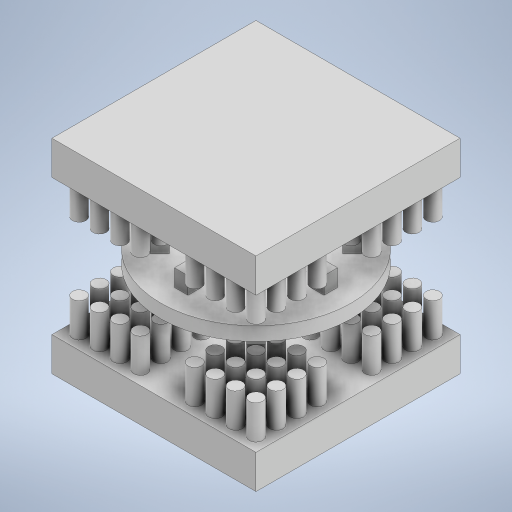
# Autodesk Inventor part: Part2
Saved by Autodesk Inventor 2024 (Build 280153000, 153)
## iProperties
Created: 2023-04-21
Part Number: Part2
Material: Generic
Document SubType Name: Modeling
Designer: Raj
Density: 1 g/cm^3
Appearance: Default
Author: Raj
Autodesk Inventor part; units mm, degrees
ref_plane "YZ Plane" through (0, 0, 0) normal (1, 0, 0) x (0, 1, 0)
ref_plane "XZ Plane" through (0, 0, 0) normal (0, 1, 0) x (-1, 0, 0)
ref_plane "XY Plane" through (0, 0, 0) normal (0, 0, 1) x (1, 0, 0)
sketch "Sketch1" plane through (0, 0, 0) normal (0, 1, 0) x (-1, 0, 0)
  point P0 (0, 0)
sketch "Sketch2" plane through (0, 0, 0) normal (0, 0, 1) x (1, 0, 0)
  line L0 (-150, 150) -> (150, 150)
  line L1 (150, 150) -> (150, -150)
  line L2 (150, -150) -> (-150, -150)
  line L3 (-150, -150) -> (-150, 150)
  line L4 (-150, 150) -> (150, -150) construction
  line L5 (150, 150) -> (-150, -150) construction
  point P0 (0, 0)
  dimension "d0" = 300
  dimension "d1" = 300
  constraints: 12 end point, 2 midpoint, 2 parallel, 1 horizontal, 1 perpendicular
  measures "d0" distance of L1.end L2.end
  measures "d1" distance of L0.end L1.end
extrude "Extrusion1" add sketch "Sketch2" along normal blind 50
sketch "Sketch3" plane through (0, 0, 50) normal (0, 0, 1) x (1, 0, 0)
  circle A0 centre (-130, -130) radius 10
  line L0 (-150, -150) -> (150, -150) projected
  line L1 (-150, 150) -> (-150, -150) projected
  circle A1 centre (-130, -100) radius 10
  circle A2 centre (-130, -70) radius 10
  circle A3 centre (-130, -40) radius 10
  circle A4 centre (-100, -130) radius 10
  circle A5 centre (-100, -100) radius 10
  circle A6 centre (-100, -70) radius 10
  circle A7 centre (-100, -40) radius 10
  circle A8 centre (-70, -130) radius 10
  circle A9 centre (-70, -100) radius 10
  circle A10 centre (-70, -70) radius 10
  circle A11 centre (-70, -40) radius 10
  circle A12 centre (-40, -130) radius 10
  circle A13 centre (-40, -100) radius 10
  circle A14 centre (-40, -70) radius 10
  circle A15 centre (-40, -40) radius 10
  circle A16 centre (-130, 130) radius 10
  line L2 (150, 150) -> (-150, 150) projected
  circle A17 centre (-100, 130) radius 10
  circle A18 centre (-70, 130) radius 10
  circle A19 centre (-40, 130) radius 10
  circle A20 centre (-130, 100) radius 10
  circle A21 centre (-100, 100) radius 10
  circle A22 centre (-70, 100) radius 10
  circle A23 centre (-40, 100) radius 10
  circle A24 centre (-130, 70) radius 10
  circle A25 centre (-100, 70) radius 10
  circle A26 centre (-70, 70) radius 10
  circle A27 centre (-40, 70) radius 10
  circle A28 centre (-130, 40) radius 10
  circle A29 centre (-100, 40) radius 10
  circle A30 centre (-70, 40) radius 10
  circle A31 centre (-40, 40) radius 10
  line L3 (0, 150) -> (0, -150) construction
  circle A32 centre (130, -130) radius 10
  circle A33 centre (130, -100) radius 10
  circle A34 centre (130, -70) radius 10
  circle A35 centre (130, -40) radius 10
  circle A36 centre (100, -130) radius 10
  circle A37 centre (100, -100) radius 10
  circle A38 centre (100, -70) radius 10
  circle A39 centre (100, -40) radius 10
  circle A40 centre (70, -130) radius 10
  circle A41 centre (70, -100) radius 10
  circle A42 centre (70, -70) radius 10
  circle A43 centre (70, -40) radius 10
  circle A44 centre (40, -130) radius 10
  circle A45 centre (40, -100) radius 10
  circle A46 centre (40, -70) radius 10
  circle A47 centre (40, -40) radius 10
  circle A48 centre (130, 130) radius 10
  circle A49 centre (100, 130) radius 10
  circle A50 centre (70, 130) radius 10
  circle A51 centre (40, 130) radius 10
  circle A52 centre (130, 100) radius 10
  circle A53 centre (100, 100) radius 10
  circle A54 centre (70, 100) radius 10
  circle A55 centre (40, 100) radius 10
  circle A56 centre (130, 70) radius 10
  circle A57 centre (100, 70) radius 10
  circle A58 centre (70, 70) radius 10
  circle A59 centre (40, 70) radius 10
  circle A60 centre (130, 40) radius 10
  circle A61 centre (100, 40) radius 10
  circle A62 centre (70, 40) radius 10
  circle A63 centre (40, 40) radius 10
  point P0 (0, 0)
  dimension "d4" = 20
  dimension "d5" = 20
  dimension "d6" = 20
  dimension "d9" = 30
  dimension "d12" = 30
  dimension "d15" = 20
  dimension "d16" = 20
  dimension "d17" = 20
  dimension "d20" = 30
  dimension "d23" = 30
  constraints: 64 centre point, 32 symmetric about line, 2 end point, 2 horizontal, 2 midpoint, 2 vertical, 92 other
  measures "d4" diameter of A0
  measures "d5" distance from line of A0.centre L0
  measures "d6" distance from line of A0.centre L1
  measures "d9" distance of A0.centre A1.centre
  measures "d12" distance of A0.centre A4.centre
  measures "d15" diameter of A16
  measures "d16" distance from line of A16.centre L2
  measures "d17" distance from line of A16.centre L1
  measures "d20" distance of A16.centre A17.centre
  measures "d23" distance of A16.centre A20.centre
extrude "Extrusion2" add sketch "Sketch3" along normal blind 50
ref_plane "Work Plane1" through (-40, -40, 150) normal (0, 0, 1) x (1, 0, 0)
sketch "Sketch4" plane through (-40, -40, 150) normal (0, 0, 1) x (1, 0, 0)
  circle A0 centre (40, 40) radius 140
  dimension "d29" = 280
  constraints: 1 centre point, 1 coincident
  measures "d29" diameter of A0
extrude "Extrusion3" add sketch "Sketch4" along normal mid plane 20
sketch "Sketch5" plane through (0, 0, 160) normal (0, 0, 1) x (1, 0, 0)
  line L0 (-110, 10) -> (-90, 10)
  line L1 (-90, 10) -> (-90, -10)
  line L2 (-90, -10) -> (-110, -10)
  line L3 (-110, -10) -> (-110, 10)
  line L4 (-110, 10) -> (-90, -10) construction
  line L5 (-90, 10) -> (-110, -10) construction
  point P0 (0, 0)
  point P1 (-100, 0)
  dimension "d32" = 20
  dimension "d33" = 20
  dimension "d34" = 100
  constraints: 12 end point, 2 midpoint, 2 parallel, 1 horizontal, 1 perpendicular
  measures "d32" distance of L1.end L2.end
  measures "d33" distance of L0.end L1.end
  measures "d34" distance of point (0, 0) point (-100, 0)
extrude "Extrusion4" add sketch "Sketch5" along normal blind 25
pattern_circular "Circular Pattern1" count 8 over 360 about axis through (0, 0, 150) along (0, 0, 1) of "Extrusion4"
mirror "Mirror1" about plane through (-40, -40, 150) normal (0, 0, 1) of "Extrusion4", "Circular Pattern1"
mirror "Mirror2" about plane through (-40, -40, 150) normal (0, 0, 1) of "Extrusion1", "Extrusion2"
body "Solid1"
